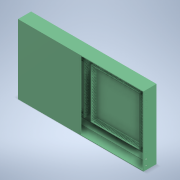
# Autodesk Inventor part: Electric Box
Saved by Autodesk Inventor 2020 (Build 240168000, 168)
## iProperties
Created: 2020-07-31
Part Number: Electric Box
Material: Generic
Document SubType Name: Modeling
Designer: Abbas
Density: 1 g/cm^3
Appearance: Default
Author: Abbas
Autodesk Inventor part; units mm, degrees
sketch "Sketch2" plane through (0, 0, 0) normal (0, 0, 1) x (1, 0, 0)
  line L0 (-110, 110) -> (110, 110)
  line L1 (110, 110) -> (110, -110)
  line L2 (110, -110) -> (-110, -110)
  line L3 (-110, -110) -> (-110, 110)
  line L4 (-110, 110) -> (110, -110) construction
  line L5 (110, 110) -> (-110, -110) construction
  line L6 (-113, 113) -> (113, 113)
  line L7 (113, 113) -> (113, -113)
  line L8 (113, -113) -> (-113, -113)
  line L9 (-113, -113) -> (-113, 113)
  line L10 (-113, 113) -> (113, -113) construction
  line L11 (113, 113) -> (-113, -113) construction
  line L12 (-366, 110) -> (-146, 110)
  line L13 (-146, 110) -> (-146, -110)
  line L14 (-146, -110) -> (-366, -110)
  line L15 (-366, -110) -> (-366, 110)
  line L16 (-366, 110) -> (-146, -110) construction
  line L17 (-146, 110) -> (-366, -110) construction
  line L18 (-369, 113) -> (-143, 113)
  line L19 (-143, 113) -> (-143, -113)
  line L20 (-143, -113) -> (-369, -113)
  line L21 (-369, -113) -> (-369, 113)
  line L22 (-369, 113) -> (-143, -113) construction
  line L23 (-143, 113) -> (-369, -113) construction
  line L24 (-143, 0) -> (-113, 0)
  line L25 (-399, 143) -> (143, 143)
  line L26 (143, 143) -> (143, -143)
  line L27 (143, -143) -> (-399, -143)
  line L28 (-399, -143) -> (-399, 143)
  line L29 (-399, 143) -> (143, -143) construction
  line L30 (143, 143) -> (-399, -143) construction
  line L31 (-402, 146) -> (146, 146)
  line L32 (146, 146) -> (146, -146)
  line L33 (146, -146) -> (-402, -146)
  line L34 (-402, -146) -> (-402, 146)
  line L35 (-402, 146) -> (146, -146) construction
  line L36 (146, 146) -> (-402, -146) construction
  line L37 (-412, 156) -> (156, 156)
  line L38 (156, 156) -> (156, -156)
  line L39 (156, -156) -> (-412, -156)
  line L40 (-412, -156) -> (-412, 156)
  line L41 (-412, 156) -> (156, -156) construction
  line L42 (156, 156) -> (-412, -156) construction
  line L43 (-415, 159) -> (159, 159)
  line L44 (159, 159) -> (159, -159)
  line L45 (159, -159) -> (-415, -159)
  line L46 (-415, -159) -> (-415, 159)
  line L47 (-415, 159) -> (159, -159) construction
  line L48 (159, 159) -> (-415, -159) construction
  point P0 (0, 0)
  point P1 (0, 0)
  point P2 (-256, 0)
  point P3 (-256, 0)
  point P4 (-128, 0)
  dimension "d21" = 220
  dimension "d22" = 220
  dimension "d23" = 226
  dimension "d24" = 226
  dimension "d25" = 220
  dimension "d26" = 220
  dimension "d27" = 226
  dimension "d28" = 226
  dimension "d29" = 30
  dimension "d30" = 542
  dimension "d31" = 286
  dimension "d32" = 548
  dimension "d33" = 292
  dimension "d34" = 568
  dimension "d35" = 312
  dimension "d36" = 574
  dimension "d37" = 318
  constraints: 98 end point, 21 midpoint, 16 parallel, 8 horizontal, 8 perpendicular
  measures "d21" distance of L1.end L2.end
  measures "d22" distance of L0.end L1.end
  measures "d23" distance of L7.end L8.end
  measures "d24" distance of L6.end L7.end
  measures "d25" distance of L13.end L14.end
  measures "d26" distance of L12.end L13.end
  measures "d27" distance of L19.end L20.end
  measures "d28" distance of L18.end L19.end
  measures "d29" distance between parallel lines of L9 L19
  measures "d30" distance of L26.end L27.end
  measures "d31" distance of L25.end L26.end
  measures "d32" distance of L32.end L33.end
  measures "d33" distance of L31.end L32.end
  measures "d34" distance of L38.end L39.end
  measures "d35" distance of L37.end L38.end
  measures "d36" distance of L44.end L45.end
  measures "d37" distance of L43.end L44.end
extrude "Extrusion1" add sketch "Sketch2" along normal blind 3 contours L0 L1 L2 L3 | L12 L13 L14 L15 | L25 L26 L27 L28 | L37 L38 L39 L40
extrude "Extrusion2" add sketch "Sketch2" along normal blind 30 contours L19 L20 L21 L18 | L6 L7 L8 L9 | L31 L32 L33 L34
extrude "Extrusion3" add sketch "Sketch2" along normal blind 60 contours L43 L44 L45 L46
sketch "Sketch3" plane through (-366, -110, 3) normal (0, 1, 0) x (1, 0, 0)
  line L0 (6, -3.5) -> (10, -3.5)
  line L1 (10, -3.5) -> (10, -23.5)
  line L2 (10, -23.5) -> (6, -23.5)
  line L3 (6, -23.5) -> (6, -3.5)
  line L4 (6, -3.5) -> (10, -23.5) construction
  line L5 (10, -3.5) -> (6, -23.5) construction
  line L6 (220, -27) -> (0, -27) projected
  line L7 (0, 0) -> (0, -27) projected
  line L8 (12, -3.5) -> (16, -3.5)
  line L9 (16, -3.5) -> (16, -23.5)
  line L10 (12, -23.5) -> (12, -3.5)
  line L11 (12, -3.5) -> (16, -23.5) construction
  line L12 (16, -3.5) -> (12, -23.5) construction
  line L13 (16, -23.5) -> (12, -23.5)
  line L14 (18, -3.5) -> (22, -3.5)
  line L15 (22, -3.5) -> (22, -23.5)
  line L16 (18, -23.5) -> (18, -3.5)
  line L17 (18, -3.5) -> (22, -23.5) construction
  line L18 (22, -3.5) -> (18, -23.5) construction
  line L19 (22, -23.5) -> (18, -23.5)
  line L20 (24, -3.5) -> (28, -3.5)
  line L21 (28, -3.5) -> (28, -23.5)
  line L22 (24, -23.5) -> (24, -3.5)
  line L23 (24, -3.5) -> (28, -23.5) construction
  line L24 (28, -3.5) -> (24, -23.5) construction
  line L25 (28, -23.5) -> (24, -23.5)
  line L26 (30, -3.5) -> (34, -3.5)
  line L27 (34, -3.5) -> (34, -23.5)
  line L28 (30, -23.5) -> (30, -3.5)
  line L29 (30, -3.5) -> (34, -23.5) construction
  line L30 (34, -3.5) -> (30, -23.5) construction
  line L31 (34, -23.5) -> (30, -23.5)
  line L32 (36, -3.5) -> (40, -3.5)
  line L33 (40, -3.5) -> (40, -23.5)
  line L34 (36, -23.5) -> (36, -3.5)
  line L35 (36, -3.5) -> (40, -23.5) construction
  line L36 (40, -3.5) -> (36, -23.5) construction
  line L37 (40, -23.5) -> (36, -23.5)
  line L38 (42, -3.5) -> (46, -3.5)
  line L39 (46, -3.5) -> (46, -23.5)
  line L40 (42, -23.5) -> (42, -3.5)
  line L41 (42, -3.5) -> (46, -23.5) construction
  line L42 (46, -3.5) -> (42, -23.5) construction
  line L43 (46, -23.5) -> (42, -23.5)
  line L44 (48, -3.5) -> (52, -3.5)
  line L45 (52, -3.5) -> (52, -23.5)
  line L46 (48, -23.5) -> (48, -3.5)
  line L47 (48, -3.5) -> (52, -23.5) construction
  line L48 (52, -3.5) -> (48, -23.5) construction
  line L49 (52, -23.5) -> (48, -23.5)
  line L50 (54, -3.5) -> (58, -3.5)
  line L51 (58, -3.5) -> (58, -23.5)
  line L52 (54, -23.5) -> (54, -3.5)
  line L53 (54, -3.5) -> (58, -23.5) construction
  line L54 (58, -3.5) -> (54, -23.5) construction
  line L55 (58, -23.5) -> (54, -23.5)
  line L56 (60, -3.5) -> (64, -3.5)
  line L57 (64, -3.5) -> (64, -23.5)
  line L58 (60, -23.5) -> (60, -3.5)
  line L59 (60, -3.5) -> (64, -23.5) construction
  line L60 (64, -3.5) -> (60, -23.5) construction
  line L61 (64, -23.5) -> (60, -23.5)
  line L62 (66, -3.5) -> (70, -3.5)
  line L63 (70, -3.5) -> (70, -23.5)
  line L64 (66, -23.5) -> (66, -3.5)
  line L65 (66, -3.5) -> (70, -23.5) construction
  line L66 (70, -3.5) -> (66, -23.5) construction
  line L67 (70, -23.5) -> (66, -23.5)
  line L68 (72, -3.5) -> (76, -3.5)
  line L69 (76, -3.5) -> (76, -23.5)
  line L70 (72, -23.5) -> (72, -3.5)
  line L71 (72, -3.5) -> (76, -23.5) construction
  line L72 (76, -3.5) -> (72, -23.5) construction
  line L73 (76, -23.5) -> (72, -23.5)
  line L74 (78, -3.5) -> (82, -3.5)
  line L75 (82, -3.5) -> (82, -23.5)
  line L76 (78, -23.5) -> (78, -3.5)
  line L77 (78, -3.5) -> (82, -23.5) construction
  line L78 (82, -3.5) -> (78, -23.5) construction
  line L79 (82, -23.5) -> (78, -23.5)
  line L80 (84, -3.5) -> (88, -3.5)
  line L81 (88, -3.5) -> (88, -23.5)
  line L82 (84, -23.5) -> (84, -3.5)
  line L83 (84, -3.5) -> (88, -23.5) construction
  line L84 (88, -3.5) -> (84, -23.5) construction
  line L85 (88, -23.5) -> (84, -23.5)
  line L86 (90, -3.5) -> (94, -3.5)
  line L87 (94, -3.5) -> (94, -23.5)
  line L88 (90, -23.5) -> (90, -3.5)
  line L89 (90, -3.5) -> (94, -23.5) construction
  line L90 (94, -3.5) -> (90, -23.5) construction
  line L91 (94, -23.5) -> (90, -23.5)
  line L92 (96, -3.5) -> (100, -3.5)
  line L93 (100, -3.5) -> (100, -23.5)
  line L94 (96, -23.5) -> (96, -3.5)
  line L95 (96, -3.5) -> (100, -23.5) construction
  line L96 (100, -3.5) -> (96, -23.5) construction
  line L97 (100, -23.5) -> (96, -23.5)
  line L98 (102, -3.5) -> (106, -3.5)
  line L99 (106, -3.5) -> (106, -23.5)
  line L100 (102, -23.5) -> (102, -3.5)
  line L101 (102, -3.5) -> (106, -23.5) construction
  line L102 (106, -3.5) -> (102, -23.5) construction
  line L103 (106, -23.5) -> (102, -23.5)
  line L104 (108, -3.5) -> (112, -3.5)
  line L105 (112, -3.5) -> (112, -23.5)
  line L106 (108, -23.5) -> (108, -3.5)
  line L107 (108, -3.5) -> (112, -23.5) construction
  line L108 (112, -3.5) -> (108, -23.5) construction
  line L109 (112, -23.5) -> (108, -23.5)
  line L110 (114, -3.5) -> (118, -3.5)
  line L111 (118, -3.5) -> (118, -23.5)
  line L112 (114, -23.5) -> (114, -3.5)
  line L113 (114, -3.5) -> (118, -23.5) construction
  line L114 (118, -3.5) -> (114, -23.5) construction
  line L115 (118, -23.5) -> (114, -23.5)
  line L116 (120, -3.5) -> (124, -3.5)
  line L117 (124, -3.5) -> (124, -23.5)
  line L118 (120, -23.5) -> (120, -3.5)
  line L119 (120, -3.5) -> (124, -23.5) construction
  line L120 (124, -3.5) -> (120, -23.5) construction
  line L121 (124, -23.5) -> (120, -23.5)
  line L122 (126, -3.5) -> (130, -3.5)
  line L123 (130, -3.5) -> (130, -23.5)
  line L124 (126, -23.5) -> (126, -3.5)
  line L125 (126, -3.5) -> (130, -23.5) construction
  line L126 (130, -3.5) -> (126, -23.5) construction
  line L127 (130, -23.5) -> (126, -23.5)
  line L128 (132, -3.5) -> (136, -3.5)
  line L129 (136, -3.5) -> (136, -23.5)
  line L130 (132, -23.5) -> (132, -3.5)
  line L131 (132, -3.5) -> (136, -23.5) construction
  line L132 (136, -3.5) -> (132, -23.5) construction
  line L133 (136, -23.5) -> (132, -23.5)
  line L134 (138, -3.5) -> (142, -3.5)
  line L135 (142, -3.5) -> (142, -23.5)
  line L136 (138, -23.5) -> (138, -3.5)
  line L137 (138, -3.5) -> (142, -23.5) construction
  line L138 (142, -3.5) -> (138, -23.5) construction
  line L139 (142, -23.5) -> (138, -23.5)
  line L140 (144, -3.5) -> (148, -3.5)
  line L141 (148, -3.5) -> (148, -23.5)
  line L142 (144, -23.5) -> (144, -3.5)
  line L143 (144, -3.5) -> (148, -23.5) construction
  line L144 (148, -3.5) -> (144, -23.5) construction
  line L145 (148, -23.5) -> (144, -23.5)
  line L146 (150, -3.5) -> (154, -3.5)
  line L147 (154, -3.5) -> (154, -23.5)
  line L148 (150, -23.5) -> (150, -3.5)
  line L149 (150, -3.5) -> (154, -23.5) construction
  line L150 (154, -3.5) -> (150, -23.5) construction
  line L151 (154, -23.5) -> (150, -23.5)
  line L152 (156, -3.5) -> (160, -3.5)
  line L153 (160, -3.5) -> (160, -23.5)
  line L154 (156, -23.5) -> (156, -3.5)
  line L155 (156, -3.5) -> (160, -23.5) construction
  line L156 (160, -3.5) -> (156, -23.5) construction
  line L157 (160, -23.5) -> (156, -23.5)
  line L158 (162, -3.5) -> (166, -3.5)
  line L159 (166, -3.5) -> (166, -23.5)
  line L160 (162, -23.5) -> (162, -3.5)
  line L161 (162, -3.5) -> (166, -23.5) construction
  line L162 (166, -3.5) -> (162, -23.5) construction
  line L163 (166, -23.5) -> (162, -23.5)
  line L164 (168, -3.5) -> (172, -3.5)
  line L165 (172, -3.5) -> (172, -23.5)
  line L166 (168, -23.5) -> (168, -3.5)
  line L167 (168, -3.5) -> (172, -23.5) construction
  line L168 (172, -3.5) -> (168, -23.5) construction
  line L169 (172, -23.5) -> (168, -23.5)
  line L170 (174, -3.5) -> (178, -3.5)
  line L171 (178, -3.5) -> (178, -23.5)
  line L172 (174, -23.5) -> (174, -3.5)
  line L173 (174, -3.5) -> (178, -23.5) construction
  line L174 (178, -3.5) -> (174, -23.5) construction
  line L175 (178, -23.5) -> (174, -23.5)
  line L176 (180, -3.5) -> (184, -3.5)
  line L177 (184, -3.5) -> (184, -23.5)
  line L178 (180, -23.5) -> (180, -3.5)
  line L179 (180, -3.5) -> (184, -23.5) construction
  line L180 (184, -3.5) -> (180, -23.5) construction
  line L181 (184, -23.5) -> (180, -23.5)
  line L182 (186, -3.5) -> (190, -3.5)
  line L183 (190, -3.5) -> (190, -23.5)
  line L184 (186, -23.5) -> (186, -3.5)
  line L185 (186, -3.5) -> (190, -23.5) construction
  line L186 (190, -3.5) -> (186, -23.5) construction
  line L187 (190, -23.5) -> (186, -23.5)
  line L188 (192, -3.5) -> (196, -3.5)
  line L189 (196, -3.5) -> (196, -23.5)
  line L190 (192, -23.5) -> (192, -3.5)
  line L191 (192, -3.5) -> (196, -23.5) construction
  line L192 (196, -3.5) -> (192, -23.5) construction
  line L193 (196, -23.5) -> (192, -23.5)
  line L194 (198, -3.5) -> (202, -3.5)
  line L195 (202, -3.5) -> (202, -23.5)
  line L196 (198, -23.5) -> (198, -3.5)
  line L197 (198, -3.5) -> (202, -23.5) construction
  line L198 (202, -3.5) -> (198, -23.5) construction
  line L199 (202, -23.5) -> (198, -23.5)
  line L200 (204, -3.5) -> (208, -3.5)
  line L201 (208, -3.5) -> (208, -23.5)
  line L202 (204, -23.5) -> (204, -3.5)
  line L203 (204, -3.5) -> (208, -23.5) construction
  line L204 (208, -3.5) -> (204, -23.5) construction
  line L205 (208, -23.5) -> (204, -23.5)
  line L206 (210, -3.5) -> (214, -3.5)
  line L207 (214, -3.5) -> (214, -23.5)
  line L208 (210, -23.5) -> (210, -3.5)
  line L209 (210, -3.5) -> (214, -23.5) construction
  line L210 (214, -3.5) -> (210, -23.5) construction
  line L211 (214, -23.5) -> (210, -23.5)
  point P0 (366, 3)
  point P1 (8, -13.5)
  point P2 (14, -13.5)
  point P3 (20, -13.5)
  point P4 (26, -13.5)
  point P5 (32, -13.5)
  point P6 (38, -13.5)
  point P7 (44, -13.5)
  point P8 (50, -13.5)
  point P9 (56, -13.5)
  point P10 (62, -13.5)
  point P11 (68, -13.5)
  point P12 (74, -13.5)
  point P13 (80, -13.5)
  point P14 (86, -13.5)
  point P15 (92, -13.5)
  point P16 (98, -13.5)
  point P17 (104, -13.5)
  point P18 (110, -13.5)
  point P19 (116, -13.5)
  point P20 (122, -13.5)
  point P21 (128, -13.5)
  point P22 (134, -13.5)
  point P23 (140, -13.5)
  point P24 (146, -13.5)
  point P25 (152, -13.5)
  point P26 (158, -13.5)
  point P27 (164, -13.5)
  point P28 (170, -13.5)
  point P29 (176, -13.5)
  point P30 (182, -13.5)
  point P31 (188, -13.5)
  point P32 (194, -13.5)
  point P33 (200, -13.5)
  point P34 (206, -13.5)
  point P35 (212, -13.5)
  dimension "d44" = 4
  dimension "d45" = 20
  dimension "d46" = 3.5
  dimension "d47" = 6
  dimension "d50" = 6
  constraints: 420 end point, 70 midpoint, 2 horizontal, 2 parallel, 1 perpendicular, 374 other
  measures "d44" distance of L1.end L2.end
  measures "d45" distance of L0.end L1.end
  measures "d46" distance between parallel lines of L6 L2
  measures "d47" distance between parallel lines of L7 L3
  measures "d50" distance of L0.start L8.start
extrude "Extrusion4" cut sketch "Sketch3" against normal blind 10
ref_plane "Work Plane1" through (-415, 0, 0) normal (0, -1, 0) x (1, 0, 0)
mirror "Mirror1" about plane through (-415, 0, 0) normal (0, -1, 0) of "Extrusion4"
ref_plane "Work Plane2" through (-128, -159, 0) normal (-1, 0, 0) x (0, 0, 1)
sketch "Sketch4" plane through (-366, -110, 3) normal (1, 0, 0) x (0, 0, -1)
  line L0 (-23.5, 214) -> (-3.5, 214)
  line L1 (-3.5, 214) -> (-3.5, 210)
  line L2 (-3.5, 210) -> (-23.5, 210)
  line L3 (-23.5, 210) -> (-23.5, 214)
  line L4 (-23.5, 214) -> (-3.5, 210) construction
  line L5 (-3.5, 214) -> (-23.5, 210) construction
  line L6 (-27, 0) -> (-27, 220) projected
  line L7 (-23.5, 208) -> (-3.5, 208)
  line L8 (-3.5, 208) -> (-3.5, 204)
  line L9 (-3.5, 204) -> (-23.5, 204)
  line L10 (-23.5, 204) -> (-23.5, 208)
  line L11 (-23.5, 208) -> (-3.5, 204) construction
  line L12 (-3.5, 208) -> (-23.5, 204) construction
  line L13 (-23.5, 202) -> (-3.5, 202)
  line L14 (-3.5, 202) -> (-3.5, 198)
  line L15 (-3.5, 198) -> (-23.5, 198)
  line L16 (-23.5, 198) -> (-23.5, 202)
  line L17 (-23.5, 202) -> (-3.5, 198) construction
  line L18 (-3.5, 202) -> (-23.5, 198) construction
  line L19 (-23.5, 196) -> (-3.5, 196)
  line L20 (-3.5, 196) -> (-3.5, 192)
  line L21 (-3.5, 192) -> (-23.5, 192)
  line L22 (-23.5, 192) -> (-23.5, 196)
  line L23 (-23.5, 196) -> (-3.5, 192) construction
  line L24 (-3.5, 196) -> (-23.5, 192) construction
  line L25 (-23.5, 190) -> (-3.5, 190)
  line L26 (-3.5, 190) -> (-3.5, 186)
  line L27 (-3.5, 186) -> (-23.5, 186)
  line L28 (-23.5, 186) -> (-23.5, 190)
  line L29 (-23.5, 190) -> (-3.5, 186) construction
  line L30 (-3.5, 190) -> (-23.5, 186) construction
  line L31 (-23.5, 184) -> (-3.5, 184)
  line L32 (-3.5, 184) -> (-3.5, 180)
  line L33 (-3.5, 180) -> (-23.5, 180)
  line L34 (-23.5, 180) -> (-23.5, 184)
  line L35 (-23.5, 184) -> (-3.5, 180) construction
  line L36 (-3.5, 184) -> (-23.5, 180) construction
  line L37 (-23.5, 178) -> (-3.5, 178)
  line L38 (-3.5, 178) -> (-3.5, 174)
  line L39 (-3.5, 174) -> (-23.5, 174)
  line L40 (-23.5, 174) -> (-23.5, 178)
  line L41 (-23.5, 178) -> (-3.5, 174) construction
  line L42 (-3.5, 178) -> (-23.5, 174) construction
  line L43 (-23.5, 172) -> (-3.5, 172)
  line L44 (-3.5, 172) -> (-3.5, 168)
  line L45 (-3.5, 168) -> (-23.5, 168)
  line L46 (-23.5, 168) -> (-23.5, 172)
  line L47 (-23.5, 172) -> (-3.5, 168) construction
  line L48 (-3.5, 172) -> (-23.5, 168) construction
  line L49 (-23.5, 166) -> (-3.5, 166)
  line L50 (-3.5, 166) -> (-3.5, 162)
  line L51 (-3.5, 162) -> (-23.5, 162)
  line L52 (-23.5, 162) -> (-23.5, 166)
  line L53 (-23.5, 166) -> (-3.5, 162) construction
  line L54 (-3.5, 166) -> (-23.5, 162) construction
  line L55 (-23.5, 160) -> (-3.5, 160)
  line L56 (-3.5, 160) -> (-3.5, 156)
  line L57 (-3.5, 156) -> (-23.5, 156)
  line L58 (-23.5, 156) -> (-23.5, 160)
  line L59 (-23.5, 160) -> (-3.5, 156) construction
  line L60 (-3.5, 160) -> (-23.5, 156) construction
  line L61 (-23.5, 154) -> (-3.5, 154)
  line L62 (-3.5, 154) -> (-3.5, 150)
  line L63 (-3.5, 150) -> (-23.5, 150)
  line L64 (-23.5, 150) -> (-23.5, 154)
  line L65 (-23.5, 154) -> (-3.5, 150) construction
  line L66 (-3.5, 154) -> (-23.5, 150) construction
  line L67 (-23.5, 148) -> (-3.5, 148)
  line L68 (-3.5, 148) -> (-3.5, 144)
  line L69 (-3.5, 144) -> (-23.5, 144)
  line L70 (-23.5, 144) -> (-23.5, 148)
  line L71 (-23.5, 148) -> (-3.5, 144) construction
  line L72 (-3.5, 148) -> (-23.5, 144) construction
  line L73 (-23.5, 142) -> (-3.5, 142)
  line L74 (-3.5, 142) -> (-3.5, 138)
  line L75 (-3.5, 138) -> (-23.5, 138)
  line L76 (-23.5, 138) -> (-23.5, 142)
  line L77 (-23.5, 142) -> (-3.5, 138) construction
  line L78 (-3.5, 142) -> (-23.5, 138) construction
  line L79 (-23.5, 136) -> (-3.5, 136)
  line L80 (-3.5, 136) -> (-3.5, 132)
  line L81 (-3.5, 132) -> (-23.5, 132)
  line L82 (-23.5, 132) -> (-23.5, 136)
  line L83 (-23.5, 136) -> (-3.5, 132) construction
  line L84 (-3.5, 136) -> (-23.5, 132) construction
  line L85 (-23.5, 130) -> (-3.5, 130)
  line L86 (-3.5, 130) -> (-3.5, 126)
  line L87 (-3.5, 126) -> (-23.5, 126)
  line L88 (-23.5, 126) -> (-23.5, 130)
  line L89 (-23.5, 130) -> (-3.5, 126) construction
  line L90 (-3.5, 130) -> (-23.5, 126) construction
  line L91 (-23.5, 124) -> (-3.5, 124)
  line L92 (-3.5, 124) -> (-3.5, 120)
  line L93 (-3.5, 120) -> (-23.5, 120)
  line L94 (-23.5, 120) -> (-23.5, 124)
  line L95 (-23.5, 124) -> (-3.5, 120) construction
  line L96 (-3.5, 124) -> (-23.5, 120) construction
  line L97 (-23.5, 118) -> (-3.5, 118)
  line L98 (-3.5, 118) -> (-3.5, 114)
  line L99 (-3.5, 114) -> (-23.5, 114)
  line L100 (-23.5, 114) -> (-23.5, 118)
  line L101 (-23.5, 118) -> (-3.5, 114) construction
  line L102 (-3.5, 118) -> (-23.5, 114) construction
  line L103 (-23.5, 112) -> (-3.5, 112)
  line L104 (-3.5, 112) -> (-3.5, 108)
  line L105 (-3.5, 108) -> (-23.5, 108)
  line L106 (-23.5, 108) -> (-23.5, 112)
  line L107 (-23.5, 112) -> (-3.5, 108) construction
  line L108 (-3.5, 112) -> (-23.5, 108) construction
  line L109 (-23.5, 106) -> (-3.5, 106)
  line L110 (-3.5, 106) -> (-3.5, 102)
  line L111 (-3.5, 102) -> (-23.5, 102)
  line L112 (-23.5, 102) -> (-23.5, 106)
  line L113 (-23.5, 106) -> (-3.5, 102) construction
  line L114 (-3.5, 106) -> (-23.5, 102) construction
  line L115 (-23.5, 100) -> (-3.5, 100)
  line L116 (-3.5, 100) -> (-3.5, 96)
  line L117 (-3.5, 96) -> (-23.5, 96)
  line L118 (-23.5, 96) -> (-23.5, 100)
  line L119 (-23.5, 100) -> (-3.5, 96) construction
  line L120 (-3.5, 100) -> (-23.5, 96) construction
  line L121 (-23.5, 94) -> (-3.5, 94)
  line L122 (-3.5, 94) -> (-3.5, 90)
  line L123 (-3.5, 90) -> (-23.5, 90)
  line L124 (-23.5, 90) -> (-23.5, 94)
  line L125 (-23.5, 94) -> (-3.5, 90) construction
  line L126 (-3.5, 94) -> (-23.5, 90) construction
  line L127 (-23.5, 88) -> (-3.5, 88)
  line L128 (-3.5, 88) -> (-3.5, 84)
  line L129 (-3.5, 84) -> (-23.5, 84)
  line L130 (-23.5, 84) -> (-23.5, 88)
  line L131 (-23.5, 88) -> (-3.5, 84) construction
  line L132 (-3.5, 88) -> (-23.5, 84) construction
  line L133 (-23.5, 82) -> (-3.5, 82)
  line L134 (-3.5, 82) -> (-3.5, 78)
  line L135 (-3.5, 78) -> (-23.5, 78)
  line L136 (-23.5, 78) -> (-23.5, 82)
  line L137 (-23.5, 82) -> (-3.5, 78) construction
  line L138 (-3.5, 82) -> (-23.5, 78) construction
  line L139 (-23.5, 76) -> (-3.5, 76)
  line L140 (-3.5, 76) -> (-3.5, 72)
  line L141 (-3.5, 72) -> (-23.5, 72)
  line L142 (-23.5, 72) -> (-23.5, 76)
  line L143 (-23.5, 76) -> (-3.5, 72) construction
  line L144 (-3.5, 76) -> (-23.5, 72) construction
  line L145 (-23.5, 70) -> (-3.5, 70)
  line L146 (-3.5, 70) -> (-3.5, 66)
  line L147 (-3.5, 66) -> (-23.5, 66)
  line L148 (-23.5, 66) -> (-23.5, 70)
  line L149 (-23.5, 70) -> (-3.5, 66) construction
  line L150 (-3.5, 70) -> (-23.5, 66) construction
  line L151 (-23.5, 64) -> (-3.5, 64)
  line L152 (-3.5, 64) -> (-3.5, 60)
  line L153 (-3.5, 60) -> (-23.5, 60)
  line L154 (-23.5, 60) -> (-23.5, 64)
  line L155 (-23.5, 64) -> (-3.5, 60) construction
  line L156 (-3.5, 64) -> (-23.5, 60) construction
  line L157 (-23.5, 58) -> (-3.5, 58)
  line L158 (-3.5, 58) -> (-3.5, 54)
  line L159 (-3.5, 54) -> (-23.5, 54)
  line L160 (-23.5, 54) -> (-23.5, 58)
  line L161 (-23.5, 58) -> (-3.5, 54) construction
  line L162 (-3.5, 58) -> (-23.5, 54) construction
  line L163 (-23.5, 52) -> (-3.5, 52)
  line L164 (-3.5, 52) -> (-3.5, 48)
  line L165 (-3.5, 48) -> (-23.5, 48)
  line L166 (-23.5, 48) -> (-23.5, 52)
  line L167 (-23.5, 52) -> (-3.5, 48) construction
  line L168 (-3.5, 52) -> (-23.5, 48) construction
  line L169 (-23.5, 46) -> (-3.5, 46)
  line L170 (-3.5, 46) -> (-3.5, 42)
  line L171 (-3.5, 42) -> (-23.5, 42)
  line L172 (-23.5, 42) -> (-23.5, 46)
  line L173 (-23.5, 46) -> (-3.5, 42) construction
  line L174 (-3.5, 46) -> (-23.5, 42) construction
  line L175 (-23.5, 40) -> (-3.5, 40)
  line L176 (-3.5, 40) -> (-3.5, 36)
  line L177 (-3.5, 36) -> (-23.5, 36)
  line L178 (-23.5, 36) -> (-23.5, 40)
  line L179 (-23.5, 40) -> (-3.5, 36) construction
  line L180 (-3.5, 40) -> (-23.5, 36) construction
  line L181 (-23.5, 34) -> (-3.5, 34)
  line L182 (-3.5, 34) -> (-3.5, 30)
  line L183 (-3.5, 30) -> (-23.5, 30)
  line L184 (-23.5, 30) -> (-23.5, 34)
  line L185 (-23.5, 34) -> (-3.5, 30) construction
  line L186 (-3.5, 34) -> (-23.5, 30) construction
  line L187 (-23.5, 28) -> (-3.5, 28)
  line L188 (-3.5, 28) -> (-3.5, 24)
  line L189 (-3.5, 24) -> (-23.5, 24)
  line L190 (-23.5, 24) -> (-23.5, 28)
  line L191 (-23.5, 28) -> (-3.5, 24) construction
  line L192 (-3.5, 28) -> (-23.5, 24) construction
  line L193 (-23.5, 22) -> (-3.5, 22)
  line L194 (-3.5, 22) -> (-3.5, 18)
  line L195 (-3.5, 18) -> (-23.5, 18)
  line L196 (-23.5, 18) -> (-23.5, 22)
  line L197 (-23.5, 22) -> (-3.5, 18) construction
  line L198 (-3.5, 22) -> (-23.5, 18) construction
  line L199 (-23.5, 16) -> (-3.5, 16)
  line L200 (-3.5, 16) -> (-3.5, 12)
  line L201 (-3.5, 12) -> (-23.5, 12)
  line L202 (-23.5, 12) -> (-23.5, 16)
  line L203 (-23.5, 16) -> (-3.5, 12) construction
  line L204 (-3.5, 16) -> (-23.5, 12) construction
  line L205 (-23.5, 10) -> (-3.5, 10)
  line L206 (-3.5, 10) -> (-3.5, 6)
  line L207 (-3.5, 6) -> (-23.5, 6)
  line L208 (-23.5, 6) -> (-23.5, 10)
  line L209 (-23.5, 10) -> (-3.5, 6) construction
  line L210 (-3.5, 10) -> (-23.5, 6) construction
  point P0 (3, 110)
  point P1 (-13.5, 212)
  point P2 (-13.5, 206)
  point P3 (-13.5, 200)
  point P4 (-13.5, 194)
  point P5 (-13.5, 188)
  point P6 (-13.5, 182)
  point P7 (-13.5, 176)
  point P8 (-13.5, 170)
  point P9 (-13.5, 164)
  point P10 (-13.5, 158)
  point P11 (-13.5, 152)
  point P12 (-13.5, 146)
  point P13 (-13.5, 140)
  point P14 (-13.5, 134)
  point P15 (-13.5, 128)
  point P16 (-13.5, 122)
  point P17 (-13.5, 116)
  point P18 (-13.5, 110)
  point P19 (-13.5, 104)
  point P20 (-13.5, 98)
  point P21 (-13.5, 92)
  point P22 (-13.5, 86)
  point P23 (-13.5, 80)
  point P24 (-13.5, 74)
  point P25 (-13.5, 68)
  point P26 (-13.5, 62)
  point P27 (-13.5, 56)
  point P28 (-13.5, 50)
  point P29 (-13.5, 44)
  point P30 (-13.5, 38)
  point P31 (-13.5, 32)
  point P32 (-13.5, 26)
  point P33 (-13.5, 20)
  point P34 (-13.5, 14)
  point P35 (-13.5, 8)
  dimension "d59" = 20
  dimension "d60" = 4
  dimension "d61" = 3.5
  dimension "d62" = 6
  dimension "d65" = 6
  constraints: 420 end point, 70 midpoint, 2 parallel, 1 horizontal, 1 perpendicular, 1 vertical, 374 other
  measures "d59" distance of L1.end L2.end
  measures "d60" distance of L0.end L1.end
  measures "d61" distance between parallel lines of L6 L3
  measures "d62" distance from line of L6.end L0
  measures "d65" distance of L0.start L7.start
extrude "Extrusion5" cut sketch "Sketch4" against normal blind 10
ref_plane "Work Plane3" through (-256, -110, 3) normal (1, 0, 0) x (0, 0, -1)
mirror "Mirror2" about plane through (-256, -110, 3) normal (1, 0, 0) of "Extrusion5"
mirror "Mirror3" about plane through (-128, -159, 0) normal (-1, 0, 0) of "Extrusion4", "Extrusion5", "Mirror1", "Mirror2"
sketch "Sketch5" plane through (0, 0, 60) normal (0, 0, 1) x (1, 0, 0)
  line L0 (-412, 156) -> (-128, 156)
  line L1 (-128, 156) -> (-128, -156)
  line L2 (-128, -156) -> (-412, -156)
  line L3 (-412, -156) -> (-412, 156)
  line L4 (-412, 156) -> (-128, -156) construction
  line L5 (-128, 156) -> (-412, -156) construction
  line L6 (-412, -156) -> (-412, 156) projected
  point P0 (0, 0)
  point P1 (-270, 0)
  point P2 (-412, 0)
  dimension "d73" = 284
  dimension "d74" = 312
  constraints: 12 end point, 4 midpoint, 2 parallel, 1 horizontal, 1 perpendicular
  measures "d73" distance of L1.end L2.end
  measures "d74" distance of L0.end L1.end
extrude "Extrusion6" add sketch "Sketch5" against normal blind 3
sketch "Sketch6" plane through (156, -156, 3) normal (-1, 0, 0) x (0, 0, 1)
  circle A0 centre (44.5, 296.989) radius 1.875
  line L0 (0, 312) -> (57, 312) projected
  circle A1 centre (44.5, 271.189) radius 1.875
  circle A2 centre (44.5, 245.389) radius 1.875
  line L1 (57, 312) -> (57, 0) projected
  point P0 (-3, 156)
  dimension "d83" = 3.75
  dimension "d85" = 15.011
  dimension "d86" = 3.75
  dimension "d87" = 3.75
  dimension "d88" = 25.8
  dimension "d89" = 25.8
  dimension "d90" = 12.5
  constraints: 3 centre point
  measures "d83" diameter of A0
  measures "d85" distance from line of L0 A0.centre
  measures "d86" diameter of A1
  measures "d87" diameter of A2
  measures "d88" distance of A1.centre A0.centre
  measures "d89" distance of A1.centre A2.centre
  measures "d90" distance from line of L1 A0.centre
extrude "Extrusion7" cut sketch "Sketch6" along normal mid plane 6
mirror "Mirror4" about plane through (-415, 0, 0) normal (0, -1, 0) of "Extrusion7"
sketch "Sketch7" plane through (0, 0, 3) normal (0, 0, 1) x (1, 0, 0)
  line L0 (-109, 1.5) -> (109, 1.5)
  line L1 (109, 1.5) -> (109, -1.5)
  line L2 (109, -1.5) -> (-109, -1.5)
  line L3 (-109, -1.5) -> (-109, 1.5)
  line L4 (-109, 1.5) -> (109, -1.5) construction
  line L5 (109, 1.5) -> (-109, -1.5) construction
  point P0 (0, 0)
  dimension "d93" = 218
  dimension "d94" = 3
  constraints: 12 end point, 2 midpoint, 2 parallel, 1 horizontal, 1 perpendicular
  measures "d93" distance of L1.end L2.end
  measures "d94" distance of L0.end L1.end
extrude "Extrusion8" add sketch "Sketch7" against normal blind 28
sketch "Sketch8" plane through (-109, -1.5, 0) normal (0, -1, 0) x (1, 0, 0)
  line L0 (218, -22) -> (0, -22)
  line L1 (0, -22) -> (0, -25)
  line L2 (0, -25) -> (218, -25)
  line L3 (218, -25) -> (218, -22)
  line L4 (218, -22) -> (0, -25) construction
  line L5 (0, -22) -> (218, -25) construction
  line L6 (218, -25) -> (0, -25) projected
  point P0 (109, 0)
  point P1 (109, -23.5)
  point P2 (109, -25)
  dimension "d97" = 218
  dimension "d98" = 3
  constraints: 12 end point, 4 midpoint, 2 parallel, 1 horizontal, 1 perpendicular
  measures "d97" distance of L2.end L1.end
  measures "d98" distance of L1.end L0.end
extrude "Extrusion9" add sketch "Sketch8" along normal blind 40
mirror "Mirror5" about plane through (-128, -159, 0) normal (-1, 0, 0) of "Extrusion9", "Extrusion8"
body "Solid1"
